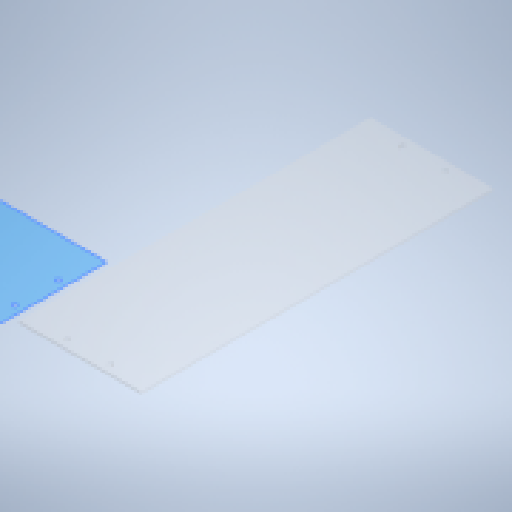
# Autodesk Inventor part: 라즈베리파이보관_윗판
Saved by Autodesk Inventor 2024 (Build 280153000, 153)
## iProperties
Created: 2024-04-10
Part Number: 라즈베리파이보관_윗판
Material: PMMA 플라스틱
Document SubType Name: Modeling
Designer: kkamin5
Mass: 91.9987 g
Surface Area: 792.88 cm^2
Volume: 77.44 cm^3
Density: 1.188 g/cm^3
Appearance: 폴리카보네이트 - 선명
Author: kkamin5
Autodesk Inventor part; units mm, degrees
ref_plane "YZ Plane" through (0, 0, 0) normal (1, 0, 0) x (0, 1, 0)
ref_plane "XZ Plane" through (0, 0, 0) normal (0, 1, 0) x (-1, 0, 0)
ref_plane "XY Plane" through (0, 0, 0) normal (0, 0, 1) x (1, 0, 0)
sketch "스케치1" plane through (0, 0, 0) normal (0, 1, 0) x (-1, 0, 0)
  line L0 (55, 195) -> (-81, 195)
  line L1 (-81, 195) -> (-81, -195)
  line L2 (-81, -195) -> (55, -195)
  line L3 (55, -195) -> (55, 195)
  point P0 (0, 0)
  dimension "d0" = 136
  dimension "d1" = 390
  dimension "d2" = 195
  dimension "d3" = 55
  constraints: 8 end point, 2 parallel, 1 horizontal, 1 perpendicular
  measures "d0" distance of L1.end L2.end
  measures "d1" distance of L0.end L1.end
  measures "d2" distance from line of point (0, 0) L2
  measures "d3" distance from line of point (0, 0) L3
extrude "돌출1" add sketch "스케치1" along normal blind 3
sketch "스케치2" plane through (0, 0, 0) normal (0, -1, 0) x (1, 0, 0)
  line L0 (81, -195) -> (-55, -195) projected
  circle A0 centre (37, -185.5) radius 2.5
  circle A1 centre (-11, -185.5) radius 2.5
  line L1 (81, 195) -> (81, -195) projected
  line L2 (46.4853, 0) -> (-31.2164, 0)
  circle A2 centre (37, 185.5) radius 2.5
  circle A3 centre (-11, 185.5) radius 2.5
  point P0 (0, 0)
  point P1 (13, -195)
  point P2 (13, -195)
  point P3 (13, 195)
  point P4 (13, 195)
  dimension "d18" = 5
  dimension "d19" = 5
  dimension "d20" = 9.5
  dimension "d21" = 0
  dimension "d22" = 48
  dimension "d23" = 44
  constraints: 4 centre point, 4 symmetric about line, 2 end point, 2 midpoint, 1 horizontal, 2 other
  measures "d18" diameter of A0
  measures "d19" diameter of A1
  measures "d20" distance from line of A0.centre L0
  measures "d21" vertical distance of A0.centre A1.centre
  measures "d22" distance of A1.centre A0.centre
  measures "d23" distance from line of L1 A0.centre
extrude "돌출2" cut sketch "스케치2" against normal blind 10
equation "\"d2\" = 0.5 * d1"
